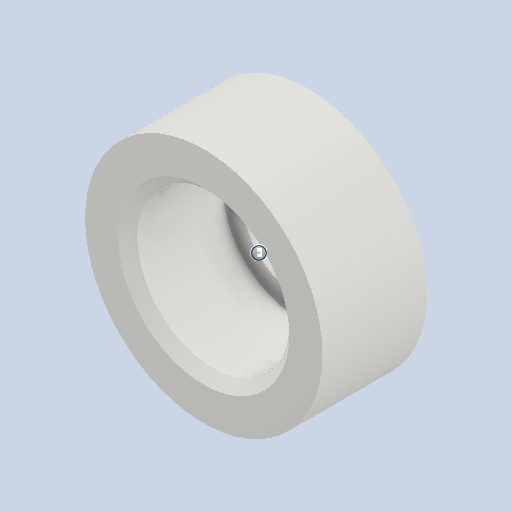
# Autodesk Inventor part: Koło pasowe zwykłe1
Saved by Autodesk Inventor 2023 (Build 270158000, 158)
## iProperties
CustomPartVersion: 1
Created: 2023-04-16
Part Number: Koło pasowe zwykłe1
Material: Steel
Document SubType Name: Modeling
Designer: krzys
Density: 7.85 g/cm^3
Appearance: Steel
Mass: 25.5103 g
Surface Area: 21.317 cm^2
Volume: 3.24972 cm^3
Author: krzys
Autodesk Inventor part; units mm, degrees
ref_plane "YZ Plane" through (0, 0, 0) normal (1, 0, 0) x (0, 1, 0)
ref_plane "XZ Plane" through (0, 0, 0) normal (0, 1, 0) x (-1, 0, 0)
ref_plane "XY Plane" through (0, 0, 0) normal (0, 0, 1) x (1, 0, 0)
sketch "Szkic główny" plane through (0, 0, 0) normal (0, 0, 1) x (1, 0, 0)
  circle A0 centre (0, 0) radius 12.5
  dimension "d0" = 25
  constraints: 1 centre point, 1 coincident
  measures "d0" diameter of A0
extrude "Koło pasowe" add sketch "Szkic główny" along normal mid plane 11
sketch "Szkic2" plane through (0, 0, 5.5) normal (0, 0, 1) x (1, 0, 0)
  circle A0 centre (0, 0) radius 8
  circle A1 centre (0, 0) radius 6
  dimension "d5" = 16
  dimension "d6" = 12
  constraints: 2 centre point, 2 coincident
  measures "d5" diameter of A0
  measures "d6" diameter of A1
extrude "Wyciągnięcie proste2" cut sketch "Szkic2" against normal through all contours A1
extrude "Wyciągnięcie proste3" cut sketch "Szkic2" against normal blind 10
chamfer "Faza1" distance 1 angle 45 1 edges at (-8, 0, 5.5)
equation "\"d0\" = da_D"
equation "\"d1\" = da_B"
equation "\"da_D\" = 25"
equation "\"da_B\" = 11"
body "Solid1"
